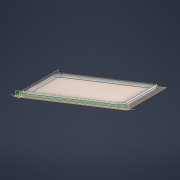
# Autodesk Inventor part: base_shape
Saved by Autodesk Inventor 2021 (Build 250183000, 183)
## iProperties
Created: 2020-09-27
Part Number: base_shape
Material: Generic
Document SubType Name: Modeling
Designer: brand
Density: 1 g/cm^3
Appearance: Default
Author: brand
Autodesk Inventor part; units mm, degrees
sketch "Sketch1" plane through (0, 0, 0) normal (0, 0, 1) x (1, 0, 0)
  line L0 (0, 0) -> (208.4, 0)
  line L1 (208.4, 0) -> (208.4, 137.5)
  line L2 (208.4, 137.5) -> (0, 137.5)
  line L3 (0, 137.5) -> (0, 0)
  dimension "d0" = 208.4
  dimension "d1" = 137.5
  constraints: 8 end point, 2 parallel, 1 horizontal, 1 perpendicular
  measures "d0" distance of L1.end L2.end
  measures "d1" distance of L0.end L1.end
extrude "Extrusion1" add sketch "Sketch1" along normal blind 7.9
fillet "Fillet1" radius 9.9 4 edges at (0, 137.5, 3.95) (0, 0, 3.95) (208.4, 0, 3.95) (208.4, 137.5, 3.95)
fillet "Fillet2" radius 2 8 edges at (205.5004, 2.8996, 7.9) (208.4, 68.75, 7.9) (205.5004, 134.6004, 7.9) (104.2, 137.5, 7.9) (2.8996, 134.6004, 7.9) (0, 68.75, 7.9) (2.8996, 2.8996, 7.9) (104.2, 0, 7.9)
fillet "Fillet3" radius 5.9 8 edges at (205.5004, 2.8996, 0) (208.4, 68.75, 0) (205.5004, 134.6004, 0) (104.2, 137.5, 0) (2.8996, 134.6004, 0) (0, 68.75, 0) (2.8996, 2.8996, 0) (104.2, 0, 0)
thicken "Thicken1" operation new thickness 0.8 both sides no extend neighbours no toward (-0.9972038, -0.0747301, 0) faces at (0.027682, 9.160172, 5.899933) (0.116105, 8.425315, 6.04946) (72.766667, 0, 5.899933) (72.766667, 0.639655, 7.366104) (202.116876, 0.68435, 5.899933) (208.283895, 8.425315, 6.04946) (208.4, 88.366667, 5.899967) (206.54946, 49.133333, 7.894408) (199.974685, 137.383895, 6.04946) (208.372318, 128.339828, 5.899933) (135.633333, 135.64946, 7.894408) (72.766667, 137.5, 5.899967) (9.160172, 137.472318, 5.899933) (8.425315, 137.383895, 6.04946) (0, 49.133333, 5.899933) (0.533896, 88.366667, 7.260345) (0.065897, 88.366667, 5.020566) (1.1046, 5.501076, 5.020566) (72.766667, 0.016497, 5.459) (202.898924, 1.1046, 5.020566) (204.655576, 49.133333, 0.407838) (207.2954, 131.998924, 5.020566) (72.766667, 133.339126, 0.262116) (1.1046, 131.998924, 5.020566) (72.766667, 89.700033, 0)
equation "\"d6\" = D - chrome_edge"
equation "\"D\" = 7.9"
equation "\"chrome_edge\" = 2"
body "Solid1"
body "Solid2"
